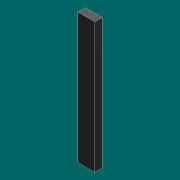
# Autodesk Inventor part: rubberizedCoating
Saved by Autodesk Inventor 2016 (Build 200138000, 138)
## iProperties
Created: 2016-02-15
Part Number: rubberizedCoating
Material: Rubber
Document SubType Name: Modeling
Designer: sawai
Density: 0.93 g/cm^3
Appearance: Rubber - Black
Author: sawai
Autodesk Inventor part; units mm, degrees
ref_plane "YZ Plane" through (0, 0, 0) normal (1, 0, 0) x (0, 1, 0)
ref_plane "XZ Plane" through (0, 0, 0) normal (0, 1, 0) x (-1, 0, 0)
ref_plane "XY Plane" through (0, 0, 0) normal (0, 0, 1) x (1, 0, 0)
sketch "Sketch1" plane through (0, 0, 0) normal (0, 0, 1) x (1, 0, 0)
  line L0 (-5.2, 5.2) -> (5.2, 5.2)
  line L1 (5.2, 5.2) -> (5.2, -5.2)
  line L2 (5.2, -5.2) -> (-5.2, -5.2)
  line L3 (-5.2, -5.2) -> (-5.2, 5.2)
  line L4 (-5.2, 5.2) -> (5.2, -5.2) construction
  line L5 (5.2, 5.2) -> (-5.2, -5.2) construction
  line L6 (5.7, 5.7) -> (-5.7, 5.7)
  line L7 (-5.7, 5.7) -> (-5.7, -5.7)
  line L8 (-5.7, -5.7) -> (5.7, -5.7)
  line L9 (5.7, -5.7) -> (5.7, 5.7)
  point P0 (0, 0)
  dimension "d0" = 10.4
  dimension "d1" = 10.4
  dimension "d2" = 0.5
  constraints: 20 end point, 4 parallel, 2 midpoint, 2 perpendicular, 1 horizontal, 3 other
  measures "d0" distance of L0.end L1.end
  measures "d1" distance between parallel lines of L3 L1
  measures "d2" distance between parallel lines of L7 L3
extrude "Extrusion1" add sketch "Sketch1" along normal blind 200.2
sketch "Sketch2" plane through (0, 0, 200.2) normal (0, 0, 1) x (1, 0, 0)
  line L0 (5.2, 5.2) -> (5.2, -5.2) projected
  line L1 (5.2, -5.2) -> (-5.2, -5.2) projected
  line L2 (-5.2, -5.2) -> (-5.2, 5.2) projected
  line L3 (-5.2, 5.2) -> (5.2, 5.2) projected
  line L4 (5.7, 5.7) -> (-5.7, 5.7) projected
  line L5 (-5.7, 5.7) -> (-5.7, -5.7) projected
  line L6 (-5.7, -5.7) -> (5.7, -5.7) projected
  line L7 (5.7, -5.7) -> (5.7, 5.7) projected
  point P0 (0, 0)
extrude "Extrusion2" add sketch "Sketch2" along normal blind 0.5 contours L0 L1 L2 L3 | L7 L6 L5 L4
equation "\"d0\" = ScintillatorThickness + 2 * silveringThickness"
equation "\"d1\" = ScintillatorWidth + 2 * silveringThickness"
equation "\"d2\" = rubberizedCoating"
equation "\"d3\" = ScintillatorHeight + silveringThickness"
equation "\"d5\" = rubberizedCoating"
equation "\"OpticalFiberClearence\" = 0.1"
equation "\"ScintillatorEdgeClearence\" = 3"
equation "\"ScintillatorHeight\" = 200"
equation "\"ShallowTrackDepth\" = 1.2"
equation "\"DeepTrackDepth\" = 5.6"
equation "\"FiberEdgeOffsett\" = 5"
equation "\"LoopLargeTrackRatio\" = 1.1"
equation "\"FiberSensorClerence\" = 0.5"
equation "\"MountingScrewOffsett\" = 9"
equation "\"silveringThickness\" = 0.2"
equation "\"rubberizedCoating\" = 0.5"
equation "\"ScintillatorThickness\" = 10"
equation "\"ScintillatorWidth\" = 10"
body "Solid1"
